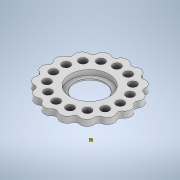
# Autodesk Inventor part: Rotor
Saved by Autodesk Inventor 2021 (Build 250183000, 183)
## iProperties
Created: 2022-07-10
Part Number: Rotor
Material: Ogólny
Document SubType Name: Modeling
Designer: MicnedSQ
Density: 1 g/cm^3
Appearance: Domyślna
Author: MicnedSQ
Autodesk Inventor part; units mm, degrees
ref_plane "YZ Plane" through (0, 0, 0) normal (1, 0, 0) x (0, 1, 0)
ref_plane "XZ Plane" through (0, 0, 0) normal (0, 1, 0) x (-1, 0, 0)
ref_plane "XY Plane" through (0, 0, 0) normal (0, 0, 1) x (1, 0, 0)
sketch "Szkic3" plane through (0, 0, 0) normal (0, 1, 0) x (-1, 0, 0)
  spline S0 degree 5 poles (31, 0) (31.0024, -0.6069) (31.1672, -1.313) (31.5398, -1.8097) (32.3428, -2.5707) (32.8903, -3.5316) (33.0734, -3.9492) (33.3819, -4.9949) (33.4301, -6.0687) (33.3732, -6.6943) (33.115, -7.84) (32.5788, -8.8868) (32.2631, -9.3517) (31.6383, -10.0507) (30.8557, -10.5934) (30.5247, -10.768) (29.3128, -11.2755) (28.3326, -12.0762) (27.8812, -13.1346) (28.0477, -14.3893) (28.4707, -15.6224) (28.5441, -15.997) (28.6392, -16.9474) (28.5017, -17.896) (28.3502, -18.4411) (27.887, -19.5373) (27.1758, -20.4715) (26.7319, -20.9191) (25.9004, -21.5568) (24.9115, -21.9922) (24.4975, -22.1133) (23.3386, -22.3337) (22.2177, -22.1974) (21.463, -22.411) (20.4034, -23.1486) (19.8086, -24.343) (19.7478, -24.9095) (19.6926, -25.9486) (19.3243, -26.9463) (19.1214, -27.3634) (18.5072, -28.2918) (17.7057, -29.0286) (17.1872, -29.3905) (16.1491, -29.926) (15.0149, -30.1858) (14.4625, -30.2446) (13.5398, -30.2153) (12.6181, -29.9713) (12.2761, -29.8214) (11.0754, -29.2677) (9.813, -29.1841) (8.7509, -29.5892) (8.0105, -30.6128) (7.362, -31.7304) (7.1131, -32.0334) (6.4441, -32.7273) (5.6117, -33.2435) (5.0908, -33.482) (3.9482, -33.8342) (2.7693, -33.8903) (2.1505, -33.8393) (1.1391, -33.617) (0.1934, -33.1506) (-0.1617, -32.9208) (-1.1047, -32.144) (-1.781, -31.1879) (-2.5967, -30.8071) (-3.861, -30.6678) (-5.1023, -31.1726) (-5.4769, -31.4988) (-6.2918, -32.0878) (-7.2339, -32.4393) (-7.708, -32.555) (-8.8198, -32.687) (-9.9259, -32.5429) (-10.531, -32.3805) (-11.6061, -31.9312) (-12.5206, -31.239) (-12.9172, -30.8613) (-13.4848, -30.1394) (-13.8977, -29.2742) (-13.9953, -28.9041) (-14.4251, -27.6471) (-15.2919, -26.7264) (-16.2996, -26.2647) (-17.5338, -26.4899) (-18.7935, -26.7176) (-19.196, -26.7222) (-20.1727, -26.658) (-21.1217, -26.3484) (-21.6482, -26.0988) (-22.6537, -25.4506) (-23.4592, -24.5786) (-23.8108, -24.0824) (-24.2882, -23.1752) (-24.5313, -22.1782) (-24.5895, -21.765) (-24.5924, -20.5158) (-24.3625, -19.3301) (-24.7474, -18.4127) (-25.5921, -17.472) (-26.8476, -17.01) (-27.2889, -16.9711) (-28.2369, -16.7155) (-29.077, -16.2531) (-29.489, -15.9474) (-30.3114, -15.1803) (-30.9254, -14.22) (-31.1881, -13.6564) (-31.5334, -12.5524) (-31.5906, -11.4207) (-31.559, -10.8877) (-31.3715, -9.9776) (-30.971, -9.0968) (-30.7326, -8.769) (-30.1445, -7.5723) (-30.1553, -6.3087) (-30.5319, -5.3148) (-31.5574, -4.6243) (-32.5306, -3.8132) (-32.8011, -3.5038) (-33.3933, -2.6979) (-33.7743, -1.7589) (-33.9248, -1.1836) (-34.0751, 0) (-33.9248, 1.1836) (-33.7743, 1.7589) (-33.3933, 2.6979) (-32.8011, 3.5038) (-32.5306, 3.8132) (-31.5574, 4.6243) (-30.5319, 5.3148) (-30.1553, 6.3087) (-30.1445, 7.5723) (-30.7326, 8.769) (-30.971, 9.0968) (-31.3715, 9.9776) (-31.559, 10.8877) (-31.5906, 11.4207) (-31.5334, 12.5524) (-31.1881, 13.6564) (-30.9254, 14.22) (-30.3114, 15.1803) (-29.489, 15.9474) (-29.077, 16.2531) (-28.2369, 16.7155) (-27.2889, 16.9711) (-26.8476, 17.01) (-25.5921, 17.472) (-24.7474, 18.4127) (-24.3625, 19.3301) (-24.5924, 20.5158) (-24.5895, 21.765) (-24.5313, 22.1782) (-24.2882, 23.1752) (-23.8108, 24.0824) (-23.4592, 24.5786) (-22.6537, 25.4506) (-21.6482, 26.0988) (-21.1217, 26.3484) (-20.1727, 26.658) (-19.196, 26.7222) (-18.7935, 26.7176) (-17.5338, 26.4899) (-16.2996, 26.2647) (-15.2919, 26.7264) (-14.4251, 27.6471) (-13.9953, 28.9041) (-13.8977, 29.2742) (-13.4848, 30.1394) (-12.9172, 30.8613) (-12.5206, 31.239) (-11.6061, 31.9312) (-10.531, 32.3805) (-9.9259, 32.5429) (-8.8198, 32.687) (-7.708, 32.555) (-7.2339, 32.4393) (-6.2918, 32.0878) (-5.4769, 31.4988) (-5.1023, 31.1726) (-3.861, 30.6678) (-2.5967, 30.8071) (-1.781, 31.1879) (-1.1047, 32.144) (-0.1617, 32.9208) (0.1934, 33.1506) (1.1391, 33.617) (2.1505, 33.8393) (2.7693, 33.8903) (3.9482, 33.8342) (5.0908, 33.482) (5.6117, 33.2435) (6.4441, 32.7273) (7.1131, 32.0334) (7.362, 31.7304) (8.0105, 30.6128) (8.7509, 29.5892) (9.813, 29.1841) (11.0754, 29.2677) (12.2761, 29.8214) (12.6181, 29.9713) (13.5398, 30.2153) (14.4625, 30.2446) (15.0149, 30.1858) (16.1491, 29.926) (17.1872, 29.3905) (17.7057, 29.0286) (18.5072, 28.2918) (19.1214, 27.3634) (19.3243, 26.9463) (19.6926, 25.9486) (19.7478, 24.9095) (19.8086, 24.343) (20.4034, 23.1486) (21.463, 22.411) (22.2177, 22.1974) (23.3386, 22.3337) (24.4975, 22.1133) (24.9115, 21.9922) (25.9004, 21.5568) (26.7319, 20.9191) (27.1758, 20.4715) (27.887, 19.5373) (28.3502, 18.4411) (28.5017, 17.896) (28.6392, 16.9474) (28.5441, 15.997) (28.4707, 15.6224) (28.0477, 14.3893) (27.8812, 13.1346) (28.3326, 12.0762) (29.3128, 11.2755) (30.5247, 10.768) (30.8557, 10.5934) (31.6383, 10.0507) (32.2631, 9.3517) (32.5788, 8.8868) (33.115, 7.84) (33.3732, 6.6943) (33.4301, 6.0687) (33.3819, 4.9949) (33.0734, 3.9492) (32.8903, 3.5316) (32.3428, 2.5707) (31.5398, 1.8097) (31.1672, 1.313) (31.0024, 0.6069) (31, 0) knots 0 0 0 0 0 0 0.013703 0.013703 0.013703 0.023651 0.023651 0.023651 0.036966 0.036966 0.036966 0.04893 0.04893 0.04893 0.057258 0.057258 0.057258 0.076735 0.076735 0.076735 0.085068 0.085068 0.085068 0.09727 0.09727 0.09727 0.110491 0.110491 0.110491 0.120135 0.120135 0.120135 0.1353 0.1353 0.1353 0.147554 0.147554 0.147554 0.15781 0.15781 0.15781 0.171195 0.171195 0.171195 0.182904 0.182904 0.182904 0.191351 0.191351 0.191351 0.210657 0.210657 0.210657 0.219088 0.219088 0.219088 0.231511 0.231511 0.231511 0.244615 0.244615 0.244615 0.253964 0.253964 0.253964 0.270446 0.270446 0.270446 0.281421 0.281421 0.281421 0.291984 0.291984 0.291984 0.305416 0.305416 0.305416 0.316856 0.316856 0.316856 0.325584 0.325584 0.325584 0.344532 0.344532 0.344532 0.353131 0.353131 0.353131 0.365754 0.365754 0.365754 0.37872 0.37872 0.37872 0.38779 0.38779 0.38779 0.405351 0.405351 0.405351 0.415308 0.415308 0.415308 0.426172 0.426172 0.426172 0.439628 0.439628 0.439628 0.450785 0.450785 0.450785 0.460002 0.460002 0.460002 0.478379 0.478379 0.478379 0.487195 0.487195 0.487195 0.5 0.5 0.5 0.512805 0.512805 0.512805 0.521621 0.521621 0.521621 0.539998 0.539998 0.539998 0.549215 0.549215 0.549215 0.560372 0.560372 0.560372 0.573828 0.573828 0.573828 0.584692 0.584692 0.584692 0.594649 0.594649 0.594649 0.61221 0.61221 0.61221 0.62128 0.62128 0.62128 0.634246 0.634246 0.634246 0.646869 0.646869 0.646869 0.655468 0.655468 0.655468 0.674416 0.674416 0.674416 0.683144 0.683144 0.683144 0.694584 0.694584 0.694584 0.708016 0.708016 0.708016 0.718579 0.718579 0.718579 0.729554 0.729554 0.729554 0.746036 0.746036 0.746036 0.755385 0.755385 0.755385 0.768489 0.768489 0.768489 0.780912 0.780912 0.780912 0.789343 0.789343 0.789343 0.808649 0.808649 0.808649 0.817096 0.817096 0.817096 0.828805 0.828805 0.828805 0.84219 0.84219 0.84219 0.852446 0.852446 0.852446 0.8647 0.8647 0.8647 0.879865 0.879865 0.879865 0.889509 0.889509 0.889509 0.90273 0.90273 0.90273 0.914932 0.914932 0.914932 0.923265 0.923265 0.923265 0.942742 0.942742 0.942742 0.95107 0.95107 0.95107 0.963034 0.963034 0.963034 0.976349 0.976349 0.976349 0.986297 0.986297 0.986297 1 1 1 1 1 1
  circle A0 centre (-25, 0) radius 3.25
  circle A1 centre (-22.8386, -10.1684) radius 3.25
  circle A2 centre (-16.7283, -18.5786) radius 3.25
  circle A3 centre (-7.7254, -23.7764) radius 3.25
  circle A4 centre (2.6132, -24.863) radius 3.25
  circle A5 centre (12.5, -21.6506) radius 3.25
  circle A6 centre (20.2254, -14.6946) radius 3.25
  circle A7 centre (24.4537, -5.1978) radius 3.25
  circle A8 centre (24.4537, 5.1978) radius 3.25
  circle A9 centre (20.2254, 14.6946) radius 3.25
  circle A10 centre (12.5, 21.6506) radius 3.25
  circle A11 centre (2.6132, 24.863) radius 3.25
  circle A12 centre (-7.7254, 23.7764) radius 3.25
  circle A13 centre (-16.7283, 18.5786) radius 3.25
  circle A14 centre (-22.8386, 10.1684) radius 3.25
  circle A15 centre (0, 0) radius 12.5
  point P0 (36, 0)
  dimension "d16" = 6.5
  dimension "d19" = 360
  dimension "d21" = 25
  dimension "d22" = 25
  constraints: 16 centre point, 1 coincident, 33 other
  measures "d16" diameter of A0
  measures "d21" distance of A0.centre point (0, 0)
  measures "d22" diameter of A15
extrude "Wyciągnięcie proste1" add sketch "Szkic3" along normal blind 5
sketch "Szkic4" plane through (0, 5, 0) normal (0, 1, 0) x (1, 0, 0)
  circle A0 centre (0, 0) radius 16
  dimension "d25" = 32
  constraints: 1 centre point, 1 coincident
  measures "d25" diameter of A0
extrude "Wyciągnięcie proste2" cut sketch "Szkic4" against normal blind 4
equation "curve S0 of \"Szkic3\": x = (35*cos(t))-(2.5*cos(t+atan(sin((1-16)*t)/((35/1.5/16)-cos((1-16)*t)))))-(1.5*cos(16*t)); y = (-35*sin(t))+(2.5*sin(t+atan(sin((1-16)*t)/((35/1.5/16)-cos((1-16)*t)))))+(1.5*s"
